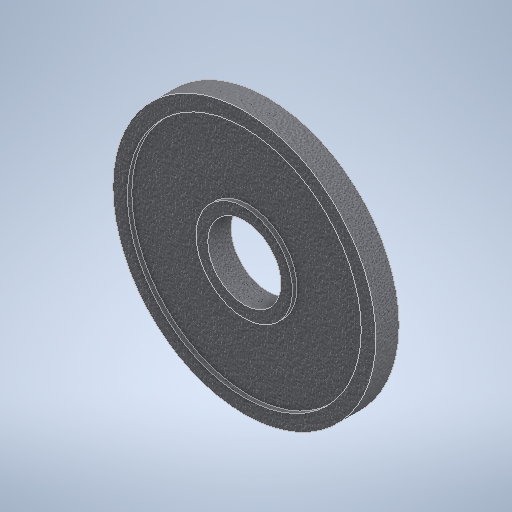
# Autodesk Inventor part: Counterweight (500g)
Saved by Autodesk Inventor 2025.2 (Build 292293000, 293)
## iProperties
Created: 2025-02-17
Part Number: Counterweight (500g)
Material: Steel, Cast
Document SubType Name: Modeling
Designer: baolo
Density: 7.85 g/cm^3
Appearance: Iron - Cast
Mass: 270.457 g
Surface Area: 156.97 cm^2
Volume: 34.4531 cm^3
Author: baolo
Autodesk Inventor part; units mm, degrees
ref_plane "YZ Plane" through (0, 0, 0) normal (1, 0, 0) x (0, 1, 0)
ref_plane "XZ Plane" through (0, 0, 0) normal (0, 1, 0) x (-1, 0, 0)
ref_plane "XY Plane" through (0, 0, 0) normal (0, 0, 1) x (1, 0, 0)
sketch "Sketch1" plane through (0, 0, 0) normal (0, 1, 0) x (-1, 0, 0)
  line L0 (16.5, 4) -> (12.5, 4)
  line L1 (12.5, 4) -> (12.5, -4)
  line L2 (12.5, -4) -> (16.5, -4)
  line L3 (16.5, -2.5) -> (40, -2.5)
  line L4 (40, 2.5) -> (16.5, 2.5)
  line L5 (40, 4) -> (45, 4)
  line L6 (45, 4) -> (45, -4)
  line L7 (45, -4) -> (40, -4)
  line L8 (16.5, 2.5) -> (16.5, 4)
  line L9 (16.5, -4) -> (16.5, -2.5)
  line L10 (40, -4) -> (40, -2.5)
  line L11 (40, 2.5) -> (40, 4)
  line L12 (0, -5.6) -> (0, 5.6) projected
  line L13 (45, 4) -> (12.5, -4) construction
  line L14 (45, -4) -> (12.5, 4) construction
  point P0 (0, 0)
  point P1 (45, 0)
  point P2 (28.75, 0)
  point P3 (40, 2)
  point P4 (16.5, -2)
  point P5 (40, -2)
  point P6 (16.5, 2)
  dimension "d1" = 90
  dimension "d2" = 5
  dimension "d3" = 4
  dimension "d4" = 25
  dimension "d5" = 8
  dimension "d7" = 1.5
  constraints: 28 end point, 7 parallel, 3 equal length, 3 horizontal, 3 midpoint, 2 horizontal alignment, 2 perpendicular
  measures "d1" diameter of L6 L12
  measures "d2" distance of L6.end L7.end
  measures "d3" distance of L1.end L2.end
  measures "d4" diameter of L1 L12
  measures "d5" distance between parallel lines of L5 L7
  measures "d7" distance between parallel lines of L3 L7
revolve "Revolution1" add sketch "Sketch1" angle 360 about axis through (0, 0, -10) along (0, 0, 1)
body "Solid1"
